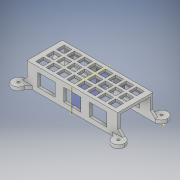
# Autodesk Inventor part: halterung_akku
Saved by Autodesk Inventor 2019 (Build 230136000, 136)
## iProperties
Created: 2018-07-23
Part Number: halterung_akku
Material: Generisch
Document SubType Name: Modeling
Designer: juliu
Density: 1 g/cm^3
Appearance: Vorgabe
Author: juliu
Autodesk Inventor part; units mm, degrees
ref_plane "YZ Plane" through (0, 0, 0) normal (1, 0, 0) x (0, 1, 0)
ref_plane "XZ Plane" through (0, 0, 0) normal (0, 1, 0) x (-1, 0, 0)
ref_plane "XY Plane" through (0, 0, 0) normal (0, 0, 1) x (1, 0, 0)
sketch "Skizze1" plane through (0, 0, 0) normal (1, 0, 0) x (0, 1, 0)
  line L0 (-20.45, 0) -> (-20.45, 26.2)
  line L1 (-20.45, 26.2) -> (20.45, 26.2)
  line L2 (20.45, 26.2) -> (20.45, 0)
  line L3 (20.45, 0) -> (17.45, 0)
  line L4 (17.45, 0) -> (17.45, 23.2)
  line L5 (17.45, 23.2) -> (-17.45, 23.2)
  line L6 (-17.45, 23.2) -> (-17.45, 0)
  line L7 (-17.45, 0) -> (-20.45, 0)
  line L8 (0, 31.44) -> (0, -5.24) projected
  line L9 (-28.63, 0) -> (28.63, 0) projected
  point P0 (0, 0)
  dimension "d0" = 34.9
  dimension "d1" = 3
  dimension "d2" = 3
  dimension "d3" = 23.2
  constraints: 16 end point, 3 perpendicular, 2 horizontal, 2 point on line, 2 vertical, 1 collinear, 1 parallel, 1 other
  measures "d0" distance between parallel lines of L4 L6
  measures "d1" distance between parallel lines of L0 L6
  measures "d2" distance between parallel lines of L1 L5
  measures "d3" distance of L3.end L4.end
extrude "Extrusion1" add sketch "Skizze1" against normal blind 130 contours L0 L1 L8 L5 L6 L7 | L1 L2 L3 L4 L5 L8
sketch "Skizze4" plane through (0, 20.45, 26.2) normal (0, 1, 0) x (1, 0, 0)
  line L0 (0, 0) -> (0, 26.2) projected
  line L1 (0, 26.2) -> (-14, 26.2)
  line L2 (-14, 26.2) -> (-14, 22.2)
  line L3 (-14, 22.2) -> (0, 22.2)
  line L4 (0, 22.2) -> (0, 26.2)
  dimension "d35" = 4
  dimension "d36" = 14
  constraints: 8 end point, 2 parallel, 1 horizontal, 1 perpendicular
  measures "d35" distance of L1.end L2.end
  measures "d36" distance of L2.end L3.end
extrude "Extrusion4" add sketch "Skizze4" along normal blind 11.55
fillet "Rundung1" radius 7 2 edges at (-14, 32, 2) (0, 32, 2)
sketch "Skizze5" plane through (-14, 20.45, 4) normal (0, 0, 1) x (1, 0, 0)
  line L0 (14, 0) -> (-116, 0) projected
  line L1 (14, 0) -> (14, 4.55) projected
  point P0 (14, -20.45)
  point P1 (7, 4.55)
  dimension "d40" = 4.55
  dimension "d41" = 7
  measures "d40" distance from line of L0 point (7, 4.55)
  measures "d41" distance from line of L1 point (7, 4.55)
hole "Bohrung1" at (-7, 25, 4) direction (0, 0, -1) diameter 3 end through all
mirror "Spiegeln1" about plane through (0, 0, 0) normal (0, 1, 0) of "Extrusion4", "Bohrung1", "Rundung1"
ref_plane "Arbeitsebene1" through (-65, 0, 0) normal (-1, 0, 0) x (0, 0, 1)
mirror "Spiegeln2" about plane through (-65, 0, 0) normal (-1, 0, 0) of "Extrusion4", "Bohrung1", "Rundung1", "Spiegeln1"
sketch "Skizze6" plane through (0, -20.45, 26.2) normal (0, 0, 1) x (1, 0, 0)
  line L0 (-27.5, 12.95) -> (-18.5, 12.95)
  line L1 (-18.5, 12.95) -> (-18.5, 3.95)
  line L2 (-18.5, 3.95) -> (-27.5, 3.95)
  line L3 (-27.5, 3.95) -> (-27.5, 12.95)
  line L4 (0, 0) -> (-130, 0) projected
  line L5 (0, 40.9) -> (0, 0) projected
  line L6 (-39.5, 12.95) -> (-30.5, 12.95)
  line L7 (-39.5, 3.95) -> (-39.5, 12.95)
  line L8 (-30.5, 12.95) -> (-30.5, 3.95)
  line L9 (-30.5, 3.95) -> (-39.5, 3.95)
  line L10 (-51.5, 12.95) -> (-42.5, 12.95)
  line L11 (-51.5, 3.95) -> (-51.5, 12.95)
  line L12 (-42.5, 12.95) -> (-42.5, 3.95)
  line L13 (-42.5, 3.95) -> (-51.5, 3.95)
  line L14 (-63.5, 12.95) -> (-54.5, 12.95)
  line L15 (-63.5, 3.95) -> (-63.5, 12.95)
  line L16 (-54.5, 12.95) -> (-54.5, 3.95)
  line L17 (-54.5, 3.95) -> (-63.5, 3.95)
  line L18 (-75.5, 12.95) -> (-66.5, 12.95)
  line L19 (-75.5, 3.95) -> (-75.5, 12.95)
  line L20 (-66.5, 12.95) -> (-66.5, 3.95)
  line L21 (-66.5, 3.95) -> (-75.5, 3.95)
  line L22 (-87.5, 12.95) -> (-78.5, 12.95)
  line L23 (-87.5, 3.95) -> (-87.5, 12.95)
  line L24 (-78.5, 12.95) -> (-78.5, 3.95)
  line L25 (-78.5, 3.95) -> (-87.5, 3.95)
  line L26 (-99.5, 12.95) -> (-90.5, 12.95)
  line L27 (-99.5, 3.95) -> (-99.5, 12.95)
  line L28 (-90.5, 12.95) -> (-90.5, 3.95)
  line L29 (-90.5, 3.95) -> (-99.5, 3.95)
  line L30 (-111.5, 12.95) -> (-102.5, 12.95)
  line L31 (-111.5, 3.95) -> (-111.5, 12.95)
  line L32 (-102.5, 12.95) -> (-102.5, 3.95)
  line L33 (-102.5, 3.95) -> (-111.5, 3.95)
  line L34 (-27.5, 24.95) -> (-18.5, 24.95)
  line L35 (-27.5, 15.95) -> (-27.5, 24.95)
  line L36 (-18.5, 24.95) -> (-18.5, 15.95)
  line L37 (-18.5, 15.95) -> (-27.5, 15.95)
  line L38 (-39.5, 24.95) -> (-30.5, 24.95)
  line L39 (-39.5, 15.95) -> (-39.5, 24.95)
  line L40 (-30.5, 24.95) -> (-30.5, 15.95)
  line L41 (-30.5, 15.95) -> (-39.5, 15.95)
  line L42 (-51.5, 24.95) -> (-42.5, 24.95)
  line L43 (-51.5, 15.95) -> (-51.5, 24.95)
  line L44 (-42.5, 24.95) -> (-42.5, 15.95)
  line L45 (-42.5, 15.95) -> (-51.5, 15.95)
  line L46 (-63.5, 24.95) -> (-54.5, 24.95)
  line L47 (-63.5, 15.95) -> (-63.5, 24.95)
  line L48 (-54.5, 24.95) -> (-54.5, 15.95)
  line L49 (-54.5, 15.95) -> (-63.5, 15.95)
  line L50 (-75.5, 24.95) -> (-66.5, 24.95)
  line L51 (-75.5, 15.95) -> (-75.5, 24.95)
  line L52 (-66.5, 24.95) -> (-66.5, 15.95)
  line L53 (-66.5, 15.95) -> (-75.5, 15.95)
  line L54 (-87.5, 24.95) -> (-78.5, 24.95)
  line L55 (-87.5, 15.95) -> (-87.5, 24.95)
  line L56 (-78.5, 24.95) -> (-78.5, 15.95)
  line L57 (-78.5, 15.95) -> (-87.5, 15.95)
  line L58 (-99.5, 24.95) -> (-90.5, 24.95)
  line L59 (-99.5, 15.95) -> (-99.5, 24.95)
  line L60 (-90.5, 24.95) -> (-90.5, 15.95)
  line L61 (-90.5, 15.95) -> (-99.5, 15.95)
  line L62 (-111.5, 24.95) -> (-102.5, 24.95)
  line L63 (-111.5, 15.95) -> (-111.5, 24.95)
  line L64 (-102.5, 24.95) -> (-102.5, 15.95)
  line L65 (-102.5, 15.95) -> (-111.5, 15.95)
  line L66 (-27.5, 36.95) -> (-18.5, 36.95)
  line L67 (-27.5, 27.95) -> (-27.5, 36.95)
  line L68 (-18.5, 36.95) -> (-18.5, 27.95)
  line L69 (-18.5, 27.95) -> (-27.5, 27.95)
  line L70 (-39.5, 36.95) -> (-30.5, 36.95)
  line L71 (-39.5, 27.95) -> (-39.5, 36.95)
  line L72 (-30.5, 36.95) -> (-30.5, 27.95)
  line L73 (-30.5, 27.95) -> (-39.5, 27.95)
  line L74 (-51.5, 36.95) -> (-42.5, 36.95)
  line L75 (-51.5, 27.95) -> (-51.5, 36.95)
  line L76 (-42.5, 36.95) -> (-42.5, 27.95)
  line L77 (-42.5, 27.95) -> (-51.5, 27.95)
  line L78 (-63.5, 36.95) -> (-54.5, 36.95)
  line L79 (-63.5, 27.95) -> (-63.5, 36.95)
  line L80 (-54.5, 36.95) -> (-54.5, 27.95)
  line L81 (-54.5, 27.95) -> (-63.5, 27.95)
  line L82 (-75.5, 36.95) -> (-66.5, 36.95)
  line L83 (-75.5, 27.95) -> (-75.5, 36.95)
  line L84 (-66.5, 36.95) -> (-66.5, 27.95)
  line L85 (-66.5, 27.95) -> (-75.5, 27.95)
  line L86 (-87.5, 36.95) -> (-78.5, 36.95)
  line L87 (-87.5, 27.95) -> (-87.5, 36.95)
  line L88 (-78.5, 36.95) -> (-78.5, 27.95)
  line L89 (-78.5, 27.95) -> (-87.5, 27.95)
  line L90 (-99.5, 36.95) -> (-90.5, 36.95)
  line L91 (-99.5, 27.95) -> (-99.5, 36.95)
  line L92 (-90.5, 36.95) -> (-90.5, 27.95)
  line L93 (-90.5, 27.95) -> (-99.5, 27.95)
  line L94 (-111.5, 36.95) -> (-102.5, 36.95)
  line L95 (-111.5, 27.95) -> (-111.5, 36.95)
  line L96 (-102.5, 36.95) -> (-102.5, 27.95)
  line L97 (-102.5, 27.95) -> (-111.5, 27.95)
  point P0 (0, 20.45)
  dimension "d73" = 9
  dimension "d74" = 9
  dimension "d75" = 3.95
  dimension "d76" = 18.5
  dimension "d79" = 12
  dimension "d82" = 12
  constraints: 192 end point, 2 horizontal, 2 parallel, 1 perpendicular, 1 vertical, 184 other
  measures "d73" distance of L0.start L0.end
  measures "d74" distance of L2.end L0.start
  measures "d75" distance between parallel lines of L4 L2
  measures "d76" distance between parallel lines of L5 L1
  measures "d79" distance of L0.start L6.start
  measures "d82" distance of L0.start L34.start
extrude "Extrusion5" cut sketch "Skizze6" against normal blind 10
sketch "Skizze7" plane through (-130, 20.45, 26.2) normal (0, 1, 0) x (1, 0, 0)
  line L0 (105, 5.6) -> (85, 5.6)
  line L1 (85, 5.6) -> (85, 20.6)
  line L2 (85, 20.6) -> (105, 20.6)
  line L3 (105, 20.6) -> (105, 5.6)
  line L4 (130, 22.2) -> (130, 0) projected
  line L5 (149.0293, 13.1) -> (50.6844, 13.1)
  line L6 (130, 0) -> (0, 0) projected
  line L7 (75, 5.6) -> (55, 5.6)
  line L8 (55, 5.6) -> (55, 20.6)
  line L9 (55, 20.6) -> (75, 20.6)
  line L10 (75, 20.6) -> (75, 5.6)
  line L11 (45, 5.6) -> (25, 5.6)
  line L12 (25, 5.6) -> (25, 20.6)
  line L13 (25, 20.6) -> (45, 20.6)
  line L14 (45, 20.6) -> (45, 5.6)
  point P0 (130, 26.2)
  dimension "d87" = 20
  dimension "d88" = 15
  dimension "d89" = 25
  dimension "d90" = 13.1
  dimension "d93" = 30
  constraints: 26 end point, 3 horizontal, 2 parallel, 1 perpendicular, 17 other
  measures "d87" distance of L0.start L0.end
  measures "d88" distance of L0.end L1.end
  measures "d89" distance between parallel lines of L4 L3
  measures "d90" distance between parallel lines of L6 L5
  measures "d93" distance of L0.start L7.start
extrude "Extrusion6" cut sketch "Skizze7" against normal through all
sketch "Skizze8" plane through (-130, 20.45, 26.2) normal (0, 1, 0) x (1, 0, 0)
  line L0 (130, 22.2) -> (130, 0) projected
  line L1 (130, 0) -> (0, 0) projected
  line L2 (130, 22.2) -> (116, 22.2) projected
  line L3 (116, 26.2) -> (14, 26.2) projected
  line L4 (130, 22.2) -> (116, 22.2) projected
  line L5 (130, 22.2) -> (130, 0)
  line L6 (130, 0) -> (117.5, 0)
  line L7 (117.5, 0) -> (117.5, 16.7)
  line L8 (117.5, 16.7) -> (123, 22.2)
  line L9 (130, 22.2) -> (123, 22.2)
  point P0 (130, 26.2)
  dimension "d100" = 12.5
  dimension "d101" = 45
  constraints: 10 end point, 2 vertical, 1 collinear, 1 midpoint, 1 point on line
  measures "d100" distance between parallel lines of L0 L7
  measures "d101" angle of L2 L8
extrude "Extrusion7" cut sketch "Skizze8" against normal through all
mirror "Spiegeln3" about plane through (-65, 0, 0) normal (-1, 0, 0) of "Extrusion7"
sketch "Skizze10" plane through (-7, 25, 4) normal (0, 0, 1) x (1, 0, 0)
  arc A0 (7, 0) -> (-7, 0) centre (0, 0) ccw projected
  line L0 (-7, 0) -> (-11.55, -4.55)
  line L1 (-7, -4.55) -> (-109, -4.55) projected
  line L2 (-7, -4.55) -> (-7, 0) projected
  line L3 (-7, -4.55) -> (-7, 0) projected
  line L4 (-7, 0) -> (-7, -4.55)
  line L5 (-7, -4.55) -> (-11.55, -4.55)
  point P0 (7, -25)
  dimension "d104" = 135
  constraints: 6 end point, 1 collinear, 1 perpendicular, 1 point on line
  measures "d104" angle of L1 L0
extrude "Extrusion8" add sketch "Skizze10" against normal blind 4
mirror "Spiegeln4" about plane through (0, 0, 0) normal (0, 1, 0) of "Extrusion8"
mirror "Spiegeln5" about plane through (-65, 0, 0) normal (-1, 0, 0) of "Extrusion8", "Spiegeln4"
sketch "Skizze11" plane through (-12.5, 20.45, 26.2) normal (0, 1, 0) x (1, 0, 0)
  point P0 (12.5, 26.2)
sketch "Skizze12" plane through (-12.5, 20.45, 26.2) normal (0, 1, 0) x (1, 0, 0)
  line L0 (0, 0) -> (-105, 0) projected
  line L1 (-105, 16.7) -> (-110.5, 22.2) projected
  line L2 (-105, 16.7) -> (-105, 0) projected
  line L3 (0, 3) -> (-105, 3) projected
  line L4 (-98.95, 3) -> (-110.5, 3)
  line L5 (-110.5, 3) -> (-110.5, 22.2)
  line L6 (-110.5, 22.2) -> (-98.95, 22.2)
  line L7 (-98.95, 22.2) -> (-98.95, 3)
  point P0 (12.5, 26.2)
  constraints: 8 end point, 2 parallel, 2 point on line, 1 horizontal, 1 perpendicular
extrude "Extrusion9" cut sketch "Skizze12" against normal blind 5 contours L1 L6 L7 L3 L2
sketch "Skizze13" plane through (-130, -25, 4) normal (0, 0, 1) x (1, 0, 0)
  line L0 (7, 7.55) -> (7, 4.55) projected
  line L1 (0, 7.55) -> (0, 0) projected
  arc A0 (7, 7.55) -> (0, 0) centre (7.5716, 0) ccw
  arc A1 (0, 0) -> (14, 0) centre (7, 0) ccw projected
  line L2 (0, 0) -> (0, 7.55)
  line L3 (0, 7.55) -> (7, 7.55)
  line L4 (130, 7.55) -> (0, 7.55) projected
  point P0 (130, 25)
  constraints: 4 end point, 2 collinear, 2 point on circle, 1 centre point, 1 tangent
extrude "Extrusion10" cut sketch "Skizze13" against normal blind 10
mirror "Spiegeln6" about plane through (0, 0, 0) normal (0, 1, 0) of "Extrusion10"
mirror "Spiegeln7" about plane through (-65, 0, 0) normal (-1, 0, 0) of "Extrusion10", "Spiegeln6"
